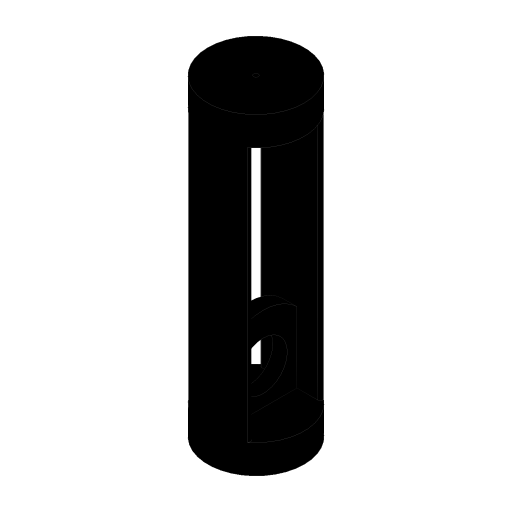
# Autodesk Inventor part: Dummy Flare
Saved by Autodesk Inventor 2024 (Build 280153000, 153)
## iProperties
Created: 2024-03-26
Part Number: Dummy Flare
Material: Generic
Document SubType Name: Modeling
Designer: Maur
Density: 1 g/cm^3
Appearance: Default
Author: Maur
Autodesk Inventor part; units mm, degrees
ref_plane "YZ Plane" through (0, 0, 0) normal (1, 0, 0) x (0, 1, 0)
ref_plane "XZ Plane" through (0, 0, 0) normal (0, 1, 0) x (-1, 0, 0)
ref_plane "XY Plane" through (0, 0, 0) normal (0, 0, 1) x (1, 0, 0)
sketch "Sketch1" plane through (0, 0, 0) normal (0, 1, 0) x (-1, 0, 0)
  circle A0 centre (0, 0) radius 20
  dimension "d0" = 40
  constraints: 1 centre point, 1 coincident
  measures "d0" diameter of A0
extrude "Extrusion1" add sketch "Sketch1" along normal blind 12
sketch "Sketch4" plane through (0, 0, 0) normal (1, 0, 0) x (0, 1, 0)
  circle A0 centre (27, 0) radius 10
  line L0 (0, -20) -> (0, 20) projected
  line L1 (12, -20) -> (12, 20) projected
  arc A1 (27, -20) -> (27, 20) centre (27, 0) ccw
  line L2 (27, 20) -> (12, 20)
  line L3 (12, -20) -> (27, -20)
  point P0 (0, 0)
  dimension "d10" = 20
  dimension "d12" = 15
  constraints: 4 end point, 2 centre point, 2 point on circle, 1 coincident, 1 horizontal, 1 tangent
  measures "d10" diameter of A0
  measures "d12" distance from line of A0.centre L1
extrude "Extrusion4" add sketch "Sketch4" along normal mid plane 6
sketch "Sketch5" plane through (0, 12, 0) normal (0, 1, 0) x (1, 0, 0)
  line L0 (15, -20) -> (-15, -20)
  line L1 (-15, -20) -> (-15, -14)
  line L2 (-15, -14) -> (15, -14)
  line L3 (15, -14) -> (15, -20)
  line L4 (3, -20) -> (3, 20) projected
  line L5 (-3, 20) -> (-3, -20) projected
  point P0 (0, 0)
  dimension "d15" = 12
  dimension "d16" = 12
  dimension "d17" = 6
  constraints: 8 end point, 2 parallel, 1 horizontal, 1 perpendicular
  measures "d15" distance between parallel lines of L4 L3
  measures "d16" distance between parallel lines of L1 L5
  measures "d17" distance between parallel lines of L0 L2
extrude "Extrusion5" add sketch "Sketch5" along normal blind 106
mirror "Mirror1" about plane through (0, 0, 0) normal (0, 0, 1) of "Extrusion5"
sketch "Sketch6" plane through (-15, 118, -20) normal (0, 1, 0) x (1, 0, 0)
  circle A0 centre (15, -20) radius 26.6667
  circle A1 centre (15, -20) radius 1
  dimension "d26" = 2
  constraints: 2 centre point, 2 coincident
  measures "d26" diameter of A1
extrude "Extrusion6" add sketch "Sketch6" along normal blind 12
sketch "Sketch7" plane through (0, 0, 0) normal (0, -1, 0) x (1, 0, 0)
  circle A0 centre (0, 0) radius 20
  circle A1 centre (0, 0) radius 37.4679
  dimension "d22" = 40
  constraints: 2 centre point, 2 coincident
  measures "d22" diameter of A0
extrude "Extrusion7" cut sketch "Sketch7" against normal through all
fillet "Fillet1" radius 1 4 edges at (-14.2829, 65, -14) (14.2829, 65, -14) (-14.2829, 65, 14) (14.2829, 65, 14)
body "Solid1"
